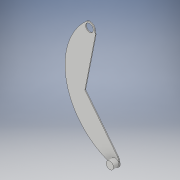
# Autodesk Inventor part: 20_Cube_Insert_CirAp_Leaf
Saved by Autodesk Inventor 2019 (Build 230136000, 136)
## iProperties
Created: 2019-10-23
Part Number: 20_Cube_Insert_CirAp_Leaf
Material: Generic
Document SubType Name: Modeling
Designer: marsikovabarbora
Density: 1 g/cm^3
Appearance: Default
Author: marsikovabarbora
Autodesk Inventor part; units mm, degrees
ref_plane "YZ Plane" through (0, 0, 0) normal (1, 0, 0) x (0, 1, 0)
ref_plane "XZ Plane" through (0, 0, 0) normal (0, 1, 0) x (-1, 0, 0)
ref_plane "XY Plane" through (0, 0, 0) normal (0, 0, 1) x (1, 0, 0)
ref_plane "Work Plane1" through (-172.2086, 28.8158, 0) normal (0, 0, 1) x (0.7311719, 0.6821933, 0)
sketch "Sketch1" plane through (-172.2086, 28.8158, 0) normal (0, 0, 1) x (0.7311719, 0.6821933, 0)
  circle A0 centre (-15.7879, -97.63) radius 1.25 construction
  circle A1 centre (-11.395, -78.3833) radius 1.25 construction
  circle A2 centre (6.3917, -69.8177) radius 1.25 construction
  arc A3 (12.3361, -69.0473) -> (8.4064, -68.3915) centre (10.3419, -68.895) ccw construction
  line L0 (8.4064, -68.3915) -> (8.3917, -68.5677) construction
  arc A4 (8.3917, -68.5677) -> (8.389, -68.4638) centre (6.3917, -68.5677) ccw construction
  arc A5 (8.389, -68.4638) -> (8.3692, -68.5658) centre (10.3419, -68.895) ccw construction
  line L1 (8.3692, -68.5658) -> (8.3837, -68.3896) construction
  arc A6 (8.3837, -68.3896) -> (4.3996, -68.3896) centre (6.3917, -68.5677) ccw construction
  line L2 (4.3996, -68.3896) -> (4.4141, -68.5658) construction
  arc A7 (4.4141, -68.5658) -> (4.3944, -68.4638) centre (2.4414, -68.895) ccw construction
  arc A8 (4.3944, -68.4638) -> (4.3917, -68.5677) centre (6.3917, -68.5677) ccw construction
  line L3 (4.3917, -68.5677) -> (4.377, -68.3915) construction
  arc A9 (4.377, -68.3915) -> (0.4472, -69.0473) centre (2.4414, -68.895) ccw construction
  line L4 (0.4472, -69.0473) -> (0.4905, -69.2186) construction
  arc A10 (0.4905, -69.2186) -> (0.4543, -69.1213) centre (-1.4011, -69.868) ccw construction
  arc A11 (0.4543, -69.1213) -> (0.4687, -69.2242) centre (2.4414, -68.895) ccw construction
  line L5 (0.4687, -69.2242) -> (0.4252, -69.0528) construction
  arc A12 (0.4252, -69.0528) -> (-3.343, -70.3465) centre (-1.4011, -69.868) ccw construction
  line L6 (-3.343, -70.3465) -> (-3.2721, -70.5084) construction
  arc A13 (-3.2721, -70.5084) -> (-3.3239, -70.4183) centre (-5.0311, -71.4603) ccw construction
  arc A14 (-3.3239, -70.4183) -> (-3.2927, -70.5174) centre (-1.4011, -69.868) ccw construction
  line L7 (-3.2927, -70.5174) -> (-3.3638, -70.3556) construction
  arc A15 (-3.3638, -70.3556) -> (-6.8678, -72.2518) centre (-5.0311, -71.4603) ccw construction
  line L8 (-6.8678, -72.2518) -> (-6.7711, -72.3999) construction
  arc A16 (-6.7711, -72.3999) -> (-6.8371, -72.3196) centre (-8.3494, -73.6283) ccw construction
  arc A17 (-6.8371, -72.3196) -> (-6.79, -72.4122) centre (-5.0311, -71.4603) ccw construction
  line L9 (-6.79, -72.4122) -> (-6.8868, -72.2642) construction
  arc A18 (-6.8868, -72.2642) -> (-10.0308, -74.7113) centre (-8.3494, -73.6283) ccw construction
  line L10 (-10.0308, -74.7113) -> (-9.9111, -74.8414) construction
  arc A19 (-9.9111, -74.8414) -> (-9.9894, -74.7731) centre (-11.2657, -76.3129) ccw construction
  arc A20 (-9.9894, -74.7731) -> (-9.9277, -74.8567) centre (-8.3494, -73.6283) ccw construction
  line L11 (-9.9277, -74.8567) -> (-10.0475, -74.7267) construction
  arc A21 (-10.0475, -74.7267) -> (-12.7459, -77.6579) centre (-11.2657, -76.3129) ccw construction
  line L12 (-12.7459, -77.6579) -> (-12.6064, -77.7666) construction
  arc A22 (-12.6064, -77.7666) -> (-12.6948, -77.712) centre (-13.7003, -79.4409) ccw construction
  arc A23 (-12.6948, -77.712) -> (-12.6203, -77.7843) centre (-11.2657, -76.3129) ccw construction
  line L13 (-12.6203, -77.7843) -> (-12.7598, -77.6758) construction
  arc A24 (-12.7598, -77.6758) -> (-14.9389, -81.0112) centre (-13.7003, -79.4409) ccw construction
  line L14 (-14.9389, -81.0112) -> (-14.7835, -81.0954) construction
  arc A25 (-14.7835, -81.0954) -> (-14.8797, -81.0562) centre (-15.5869, -82.927) ccw construction
  arc A26 (-14.8797, -81.0562) -> (-14.7942, -81.1152) centre (-13.7003, -79.4409) ccw construction
  line L15 (-14.7942, -81.1152) -> (-14.9497, -81.0312) construction
  arc A27 (-14.9497, -81.0312) -> (-16.5501, -84.6797) centre (-15.5869, -82.927) ccw construction
  line L16 (-16.5501, -84.6797) -> (-16.383, -84.7372) construction
  arc A28 (-16.383, -84.7372) -> (-16.4843, -84.7143) centre (-16.8739, -86.676) ccw construction
  arc A29 (-16.4843, -84.7143) -> (-16.3903, -84.7585) centre (-15.5869, -82.927) ccw construction
  line L17 (-16.3903, -84.7585) -> (-16.5575, -84.7012) construction
  arc A30 (-16.5575, -84.7012) -> (-17.5355, -88.5634) centre (-16.8739, -86.676) ccw construction
  line L18 (-17.5355, -88.5634) -> (-17.3612, -88.5926) construction
  arc A31 (-17.3612, -88.5926) -> (-17.4649, -88.5867) centre (-17.5264, -90.5857) ccw construction
  arc A32 (-17.4649, -88.5867) -> (-17.3649, -88.6148) centre (-16.8739, -86.676) ccw construction
  line L19 (-17.3649, -88.6148) -> (-17.5393, -88.5858) construction
  arc A33 (-17.5393, -88.5858) -> (-17.8683, -92.5563) centre (-17.5264, -90.5857) ccw construction
  line L20 (-17.8683, -92.5563) -> (-17.6915, -92.5564) construction
  arc A34 (-17.6915, -92.5564) -> (-17.7948, -92.5677) centre (-17.5264, -94.5496) ccw construction
  arc A35 (-17.7948, -92.5677) -> (-17.6915, -92.5789) centre (-17.5264, -90.5857) ccw construction
  line L21 (-17.6915, -92.5789) -> (-17.8683, -92.579) construction
  arc A36 (-17.8683, -92.579) -> (-17.5393, -96.5495) centre (-17.5264, -94.5496) ccw construction
  line L22 (-17.5393, -96.5495) -> (-17.3649, -96.5205) construction
  arc A37 (-17.3649, -96.5205) -> (-17.4649, -96.5486) centre (-16.8739, -98.4593) ccw construction
  arc A38 (-17.4649, -96.5486) -> (-17.3612, -96.5427) centre (-17.5264, -94.5496) ccw construction
  line L23 (-17.3612, -96.5427) -> (-17.5355, -96.5719) construction
  arc A39 (-17.5355, -96.5719) -> (-16.5575, -100.4341) centre (-16.8739, -98.4593) ccw construction
  line L24 (-16.5575, -100.4341) -> (-16.3903, -100.3768) construction
  arc A40 (-16.3903, -100.3768) -> (-16.4843, -100.421) centre (-15.5869, -102.2083) ccw construction
  arc A41 (-16.4843, -100.421) -> (-16.383, -100.3981) centre (-16.8739, -98.4593) ccw construction
  line L25 (-16.383, -100.3981) -> (-16.5501, -100.4556) construction
  arc A42 (-16.5501, -100.4556) -> (-14.9497, -104.1041) centre (-15.5869, -102.2083) ccw construction
  line L26 (-14.9497, -104.1041) -> (-14.7942, -104.0201) construction
  arc A43 (-14.7942, -104.0201) -> (-14.8797, -104.0791) centre (-13.7003, -105.6944) ccw construction
  arc A44 (-14.8797, -104.0791) -> (-14.7835, -104.0399) centre (-15.5869, -102.2083) ccw construction
  line L27 (-14.7835, -104.0399) -> (-14.9389, -104.1241) construction
  arc A45 (-14.9389, -104.1241) -> (-12.7598, -107.4595) centre (-13.7003, -105.6944) ccw construction
  line L28 (-12.7598, -107.4595) -> (-12.6203, -107.351) construction
  arc A46 (-12.6203, -107.351) -> (-12.6948, -107.4233) centre (-11.2657, -108.8224) ccw construction
  arc A47 (-12.6948, -107.4233) -> (-12.6064, -107.3687) centre (-13.7003, -105.6944) ccw construction
  line L29 (-12.6064, -107.3687) -> (-12.7459, -107.4774) construction
  arc A48 (-12.7459, -107.4774) -> (-10.0475, -110.4086) centre (-11.2657, -108.8224) ccw construction
  line L30 (-10.0475, -110.4086) -> (-9.9277, -110.2786) construction
  arc A49 (-9.9277, -110.2786) -> (-9.9894, -110.3622) centre (-8.3494, -111.507) ccw construction
  arc A50 (-9.9894, -110.3622) -> (-9.9111, -110.2939) centre (-11.2657, -108.8224) ccw construction
  line L31 (-9.9111, -110.2939) -> (-10.0308, -110.424) construction
  arc A51 (-10.0308, -110.424) -> (-6.8868, -112.8711) centre (-8.3494, -111.507) ccw construction
  line L32 (-6.8868, -112.8711) -> (-6.79, -112.7231) construction
  arc A52 (-6.79, -112.7231) -> (-6.8371, -112.8157) centre (-5.0311, -113.675) ccw construction
  arc A53 (-6.8371, -112.8157) -> (-6.7711, -112.7355) centre (-8.3494, -111.507) ccw construction
  line L33 (-6.7711, -112.7355) -> (-6.8678, -112.8835) construction
  arc A54 (-6.8678, -112.8835) -> (-3.3638, -114.7797) centre (-5.0311, -113.675) ccw construction
  line L34 (-3.3638, -114.7797) -> (-3.2927, -114.6179) construction
  arc A55 (-3.2927, -114.6179) -> (-3.3239, -114.717) centre (-1.4011, -115.2673) ccw construction
  arc A56 (-3.3239, -114.717) -> (-3.2721, -114.6269) centre (-5.0311, -113.675) ccw construction
  line L35 (-3.2721, -114.6269) -> (-3.343, -114.7888) construction
  arc A57 (-3.343, -114.7888) -> (0.4252, -116.0825) centre (-1.4011, -115.2673) ccw construction
  line L36 (0.4252, -116.0825) -> (0.4687, -115.9111) construction
  arc A58 (0.4687, -115.9111) -> (0.4543, -116.014) centre (2.4414, -116.2403) ccw construction
  arc A59 (0.4543, -116.014) -> (0.4905, -115.9167) centre (-1.4011, -115.2673) ccw construction
  line L37 (0.4905, -115.9167) -> (0.4472, -116.088) construction
  arc A60 (0.4472, -116.088) -> (4.377, -116.7438) centre (2.4414, -116.2403) ccw construction
  line L38 (4.377, -116.7438) -> (4.3917, -116.5677) construction
  arc A61 (4.3917, -116.5677) -> (4.3944, -116.6715) centre (6.3917, -116.5677) ccw construction
  arc A62 (4.3944, -116.6715) -> (4.4141, -116.5695) centre (2.4414, -116.2403) ccw construction
  line L39 (4.4141, -116.5695) -> (4.3996, -116.7457) construction
  arc A63 (4.3996, -116.7457) -> (8.3837, -116.7457) centre (6.3917, -116.5677) ccw construction
  line L40 (8.3837, -116.7457) -> (8.3692, -116.5695) construction
  arc A64 (8.3692, -116.5695) -> (8.389, -116.6715) centre (10.3419, -116.2403) ccw construction
  arc A65 (8.389, -116.6715) -> (8.3917, -116.5677) centre (6.3917, -116.5677) ccw construction
  line L41 (8.3917, -116.5677) -> (8.4064, -116.7438) construction
  arc A66 (8.4064, -116.7438) -> (12.3361, -116.088) centre (10.3419, -116.2403) ccw construction
  line L42 (12.3361, -116.088) -> (12.2928, -115.9167) construction
  arc A67 (12.2928, -115.9167) -> (12.3291, -116.014) centre (14.1845, -115.2673) ccw construction
  arc A68 (12.3291, -116.014) -> (12.3147, -115.9111) centre (10.3419, -116.2403) ccw construction
  line L43 (12.3147, -115.9111) -> (12.3581, -116.0825) construction
  arc A69 (12.3581, -116.0825) -> (16.1264, -114.7888) centre (14.1845, -115.2673) ccw construction
  line L44 (16.1264, -114.7888) -> (16.0555, -114.6269) construction
  arc A70 (16.0555, -114.6269) -> (16.1073, -114.717) centre (17.8144, -113.675) ccw construction
  arc A71 (16.1073, -114.717) -> (16.0761, -114.6179) centre (14.1845, -115.2673) ccw construction
  line L45 (16.0761, -114.6179) -> (16.1472, -114.7797) construction
  arc A72 (16.1472, -114.7797) -> (19.6511, -112.8835) centre (17.8144, -113.675) ccw construction
  line L46 (19.6511, -112.8835) -> (19.5545, -112.7355) construction
  arc A73 (19.5545, -112.7355) -> (19.6204, -112.8157) centre (21.1328, -111.507) ccw construction
  arc A74 (19.6204, -112.8157) -> (19.5734, -112.7231) centre (17.8144, -113.675) ccw construction
  line L47 (19.5734, -112.7231) -> (19.6701, -112.8711) construction
  arc A75 (19.6701, -112.8711) -> (22.8141, -110.424) centre (21.1328, -111.507) ccw construction
  line L48 (22.8141, -110.424) -> (22.6945, -110.2939) construction
  arc A76 (22.6945, -110.2939) -> (22.7727, -110.3622) centre (24.049, -108.8224) ccw construction
  arc A77 (22.7727, -110.3622) -> (22.7111, -110.2786) centre (21.1328, -111.507) ccw construction
  line L49 (22.7111, -110.2786) -> (22.8308, -110.4086) construction
  arc A78 (22.8308, -110.4086) -> (25.5292, -107.4774) centre (24.049, -108.8224) ccw construction
  line L50 (25.5292, -107.4774) -> (25.3898, -107.3687) construction
  arc A79 (25.3898, -107.3687) -> (25.4782, -107.4233) centre (26.4837, -105.6944) ccw construction
  arc A80 (25.4782, -107.4233) -> (25.4036, -107.351) centre (24.049, -108.8224) ccw construction
  line L51 (25.4036, -107.351) -> (25.5431, -107.4595) construction
  arc A81 (25.5431, -107.4595) -> (27.7223, -104.1241) centre (26.4837, -105.6944) ccw construction
  line L52 (27.7223, -104.1241) -> (27.5668, -104.0399) construction
  arc A82 (27.5668, -104.0399) -> (27.663, -104.0791) centre (28.3702, -102.2083) ccw construction
  arc A83 (27.663, -104.0791) -> (27.5776, -104.0201) centre (26.4837, -105.6944) ccw construction
  line L53 (27.5776, -104.0201) -> (27.7331, -104.1041) construction
  arc A84 (27.7331, -104.1041) -> (29.3335, -100.4556) centre (28.3702, -102.2083) ccw construction
  line L54 (29.3335, -100.4556) -> (29.1663, -100.3981) construction
  arc A85 (29.1663, -100.3981) -> (29.2676, -100.421) centre (29.6573, -98.4593) ccw construction
  arc A86 (29.2676, -100.421) -> (29.1736, -100.3768) centre (28.3702, -102.2083) ccw construction
  line L55 (29.1736, -100.3768) -> (29.3408, -100.4341) construction
  arc A87 (29.3408, -100.4341) -> (30.3189, -96.5719) centre (29.6573, -98.4593) ccw construction
  line L56 (30.3189, -96.5719) -> (30.1445, -96.5427) construction
  arc A88 (30.1445, -96.5427) -> (30.2483, -96.5486) centre (30.3097, -94.5496) ccw construction
  arc A89 (30.2483, -96.5486) -> (30.1483, -96.5205) centre (29.6573, -98.4593) ccw construction
  line L57 (30.1483, -96.5205) -> (30.3226, -96.5495) construction
  arc A90 (30.3226, -96.5495) -> (30.6516, -92.579) centre (30.3097, -94.5496) ccw construction
  line L58 (30.6516, -92.579) -> (30.4749, -92.5789) construction
  arc A91 (30.4749, -92.5789) -> (30.5781, -92.5677) centre (30.3097, -90.5857) ccw construction
  arc A92 (30.5781, -92.5677) -> (30.4749, -92.5564) centre (30.3097, -94.5496) ccw construction
  line L59 (30.4749, -92.5564) -> (30.6516, -92.5563) construction
  arc A93 (30.6516, -92.5563) -> (30.3226, -88.5858) centre (30.3097, -90.5857) ccw construction
  line L60 (30.3226, -88.5858) -> (30.1483, -88.6148) construction
  arc A94 (30.1483, -88.6148) -> (30.2483, -88.5867) centre (29.6573, -86.676) ccw construction
  arc A95 (30.2483, -88.5867) -> (30.1445, -88.5926) centre (30.3097, -90.5857) ccw construction
  line L61 (30.1445, -88.5926) -> (30.3189, -88.5634) construction
  arc A96 (30.3189, -88.5634) -> (29.3408, -84.7012) centre (29.6573, -86.676) ccw construction
  line L62 (29.3408, -84.7012) -> (29.1736, -84.7585) construction
  arc A97 (29.1736, -84.7585) -> (29.2676, -84.7143) centre (28.3702, -82.927) ccw construction
  arc A98 (29.2676, -84.7143) -> (29.1663, -84.7372) centre (29.6573, -86.676) ccw construction
  line L63 (29.1663, -84.7372) -> (29.3335, -84.6797) construction
  arc A99 (29.3335, -84.6797) -> (27.7331, -81.0312) centre (28.3702, -82.927) ccw construction
  line L64 (27.7331, -81.0312) -> (27.5776, -81.1152) construction
  arc A100 (27.5776, -81.1152) -> (27.663, -81.0562) centre (26.4837, -79.4409) ccw construction
  arc A101 (27.663, -81.0562) -> (27.5668, -81.0954) centre (28.3702, -82.927) ccw construction
  line L65 (27.5668, -81.0954) -> (27.7223, -81.0112) construction
  arc A102 (27.7223, -81.0112) -> (25.5431, -77.6758) centre (26.4837, -79.4409) ccw construction
  line L66 (25.5431, -77.6758) -> (25.4036, -77.7843) construction
  arc A103 (25.4036, -77.7843) -> (25.4782, -77.712) centre (24.049, -76.3129) ccw construction
  arc A104 (25.4782, -77.712) -> (25.3898, -77.7666) centre (26.4837, -79.4409) ccw construction
  line L67 (25.3898, -77.7666) -> (25.5292, -77.6579) construction
  arc A105 (25.5292, -77.6579) -> (22.8308, -74.7267) centre (24.049, -76.3129) ccw construction
  line L68 (22.8308, -74.7267) -> (22.7111, -74.8567) construction
  arc A106 (22.7111, -74.8567) -> (22.7727, -74.7731) centre (21.1328, -73.6283) ccw construction
  arc A107 (22.7727, -74.7731) -> (22.6945, -74.8414) centre (24.049, -76.3129) ccw construction
  line L69 (22.6945, -74.8414) -> (22.8141, -74.7113) construction
  arc A108 (22.8141, -74.7113) -> (19.6701, -72.2642) centre (21.1328, -73.6283) ccw construction
  line L70 (19.6701, -72.2642) -> (19.5734, -72.4122) construction
  arc A109 (19.5734, -72.4122) -> (19.6204, -72.3196) centre (17.8144, -71.4603) ccw construction
  arc A110 (19.6204, -72.3196) -> (19.5545, -72.3999) centre (21.1328, -73.6283) ccw construction
  line L71 (19.5545, -72.3999) -> (19.6511, -72.2518) construction
  arc A111 (19.6511, -72.2518) -> (16.1472, -70.3556) centre (17.8144, -71.4603) ccw construction
  line L72 (16.1472, -70.3556) -> (16.0761, -70.5174) construction
  arc A112 (16.0761, -70.5174) -> (16.1073, -70.4183) centre (14.1845, -69.868) ccw construction
  arc A113 (16.1073, -70.4183) -> (16.0555, -70.5084) centre (17.8144, -71.4603) ccw construction
  line L73 (16.0555, -70.5084) -> (16.1264, -70.3465) construction
  arc A114 (16.1264, -70.3465) -> (12.3581, -69.0528) centre (14.1845, -69.868) ccw construction
  line L74 (12.3581, -69.0528) -> (12.3147, -69.2242) construction
  arc A115 (12.3147, -69.2242) -> (12.3291, -69.1213) centre (10.3419, -68.895) ccw construction
  arc A116 (12.3291, -69.1213) -> (12.2928, -69.2186) centre (14.1845, -69.868) ccw construction
  line L75 (12.2928, -69.2186) -> (12.3361, -69.0473) construction
  circle A117 centre (6.3917, -92.5677) radius 21 construction
  circle A118 centre (-13.1155, -104.9383) radius 1.4
  arc A119 (6.4025, -67.85) -> (-14.4494, -105.8573) centre (6.3917, -92.5677) ccw
  circle A120 centre (6.3917, -69.8177) radius 1.45
  arc A121 (7.7753, -71.2167) -> (6.4025, -67.85) centre (6.3917, -69.8177) ccw
  line L76 (6.3917, -69.8177) -> (7.7753, -71.2167) construction
  line L77 (6.3917, -69.8177) -> (6.4025, -67.85) construction
  arc A122 (-14.5155, -105.753) -> (-11.5494, -105.3521) centre (-13.1155, -104.9383) ccw
  line L78 (-13.1155, -104.9383) -> (-11.5494, -105.3521) construction
  line L79 (-13.1155, -104.9383) -> (-14.5155, -105.753) construction
  line L80 (-11.5494, -105.3521) -> (7.7753, -71.2167)
  circle A123 centre (24.1783, -78.3833) radius 1.25
  circle A124 centre (28.5713, -97.63) radius 1.25
  circle A125 centre (16.2625, -113.0647) radius 1.25
  circle A126 centre (-3.4792, -113.0647) radius 1.25
  point P0 (106.2561, -138.5489)
  dimension "d0" = 2.8
  dimension "d1" = 0.2
  dimension "d2" = 135
  dimension "d3" = 135
  constraints: 236 point on circle, 162 end point, 127 centre point, 3 coincident, 4 other
  measures "d0" diameter of A118
  measures "d1" radial gap between concentric circles of A2 A120
  measures "d2" angle of L76 L77
  measures "d3" angle of L79 L78
extrude "Extrusion1" add sketch "Sketch1" along normal blind 0.3 contours A118 | A121 L80 A122 A119
sketch "Sketch2" plane through (-172.2086, 28.8158, 0.3) normal (0, 0, 1) x (0.7311719, 0.6821933, 0)
  circle A0 centre (6.3917, -69.8177) radius 1.45 construction
  arc A1 (6.4025, -67.85) -> (-14.4494, -105.8573) centre (6.3917, -92.5677) ccw construction
  arc A2 (-14.4494, -105.8573) -> (-11.5494, -105.3521) centre (-13.1155, -104.9383) ccw construction
  line L0 (-11.5494, -105.3521) -> (7.7753, -71.2167) construction
  arc A3 (7.7753, -71.2167) -> (6.4025, -67.85) centre (6.3917, -69.8177) ccw construction
  circle A4 centre (-13.1155, -104.9383) radius 1.4
  point P0 (106.2561, -138.5489)
  dimension "d6" = 2.8
  constraints: 1 centre point, 1 coincident
  measures "d6" diameter of A4
extrude "Extrusion2" add sketch "Sketch2" along normal blind 2
sketch "Sketch3" plane through (-172.2086, 28.8158, 0.3) normal (0, 0, 1) x (0.7311719, 0.6821933, 0)
  circle A0 centre (-13.1155, -104.9383) radius 1.4 construction
  circle A1 centre (6.3917, -69.8177) radius 1.45 construction
  arc A2 (6.4025, -67.85) -> (-14.4494, -105.8573) centre (6.3917, -92.5677) ccw construction
  arc A3 (-14.4494, -105.8573) -> (-11.5494, -105.3521) centre (-13.1155, -104.9383) ccw construction
  line L0 (-11.5494, -105.3521) -> (7.7753, -71.2167) construction
  arc A4 (7.7753, -71.2167) -> (6.4025, -67.85) centre (6.3917, -69.8177) ccw construction
  line L1 (-11.5494, -105.3521) -> (7.7753, -71.2167) construction
  line L2 (-1.887, -88.2844) -> (-15.2891, -80.6972) construction
  line L3 (-9.284, -84.0968) -> (7.2157, -72.2053)
  line L4 (-9.284, -84.0968) -> (-10.9897, -104.3635)
  line L5 (-10.9897, -104.3635) -> (7.2157, -72.2053)
  point P0 (106.2561, -138.5489)
  dimension "d20" = 8.5
  constraints: 8 end point, 2 point on line, 1 collinear, 1 midpoint, 1 perpendicular, 1 point on circle, 1 symmetric about line
  measures "d20" distance from line of L0 L3.start
extrude "Extrusion3" cut sketch "Sketch3" against normal through all
fillet "Fillet1" radius 2 2 edges at (-109.048, -54.9889, 0.15) (-117.6748, -19.0562, 0.15)
sketch "Sketch4" plane through (-172.2086, 28.8158, 0.3) normal (0, 0, 1) x (0.7311719, 0.6821933, 0)
  line L0 (7.4314, -71.8242) -> (7.7753, -71.2167) construction
  arc A0 (7.7753, -71.2167) -> (6.4025, -67.85) centre (6.3917, -69.8177) ccw construction
  arc A1 (6.4025, -67.85) -> (-14.4494, -105.8573) centre (6.3917, -92.5677) ccw construction
  arc A2 (-14.4494, -105.8573) -> (-11.5494, -105.3521) centre (-13.1155, -104.9383) ccw construction
  circle A3 centre (-13.1155, -104.9383) radius 1.4 construction
  circle A4 centre (6.3917, -69.8177) radius 1.45 construction
  line L1 (-20.7146, -92.3351) -> (-11.0435, -83.146)
  line L2 (-10.953, -103.9271) -> (-9.284, -84.0968) projected
  line L3 (6.3917, -92.5677) -> (-12.496, -82.3611) construction
  line L4 (-9.284, -84.0968) -> (6.8604, -72.4614) construction
  line L5 (-20.7146, -92.3351) -> (-9.284, -84.0968)
  line L6 (-11.0435, -83.146) -> (-5.8817, -43.6741)
  line L7 (-9.284, -84.0968) -> (-5.8817, -43.6741)
  arc A5 (6.8604, -72.4614) -> (7.4314, -71.8242) centre (5.691, -70.8389) ccw projected
  line L8 (-11.5494, -105.3521) -> (-11.2055, -104.7446) projected
  arc A6 (-11.2055, -104.7446) -> (-10.953, -103.9271) centre (-12.946, -103.7593) ccw projected
  line L9 (-10.953, -103.9271) -> (-9.284, -84.0968) projected
  line L10 (-9.284, -84.0968) -> (6.8604, -72.4614) projected
  point P0 (106.2561, -138.5489)
  point P1 (-16.9547, -84.4492)
  point P2 (-13.1031, -77.3717)
  dimension "d12" = 2
  constraints: 10 end point, 2 point on line, 5 other
  measures "d12" distance of L5.end L1.end
extrude "Extrusion4" [suppressed]
sketch "Sketch5" plane through (-172.2086, 28.8158, 0.3) normal (0, 0, 1) x (0.7311719, 0.6821933, 0)
  line L0 (7.4314, -71.8242) -> (7.7753, -71.2167) projected
  arc A0 (7.7753, -71.2167) -> (6.4025, -67.85) centre (6.3917, -69.8177) ccw projected
  arc A1 (6.4025, -67.85) -> (-14.4494, -105.8573) centre (6.3917, -92.5677) ccw projected
  arc A2 (-14.4494, -105.8573) -> (-11.5494, -105.3521) centre (-13.1155, -104.9383) ccw projected
  circle A3 centre (-13.1155, -104.9383) radius 1.4 projected
  circle A4 centre (6.3917, -69.8177) radius 1.45 projected
  line L1 (7.4314, -71.8242) -> (7.7753, -71.2167) projected
  line L2 (-11.5494, -105.3521) -> (-11.2055, -104.7446) projected
  arc A5 (7.1804, -72.1737) -> (-11.2055, -104.7446) centre (1.7027, -90.5564) ccw
  line L3 (7.1804, -72.1737) -> (-11.2055, -104.7446)
  arc A6 (6.8604, -72.4614) -> (7.4314, -71.8242) centre (5.691, -70.8389) ccw projected
  line L4 (-11.5494, -105.3521) -> (-11.2055, -104.7446) projected
  arc A7 (-11.2055, -104.7446) -> (-10.953, -103.9271) centre (-12.946, -103.7593) ccw projected
  line L5 (-10.953, -103.9271) -> (-9.284, -84.0968) projected
  line L6 (-9.284, -84.0968) -> (6.8604, -72.4614) projected
  point P0 (106.2561, -138.5489)
  constraints: 4 point on circle, 2 end point, 1 centre point
extrude "Extrusion5" [suppressed]
body "Solid1"
